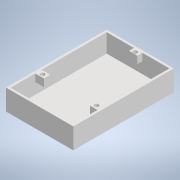
# Autodesk Inventor part: корпус
Saved by Autodesk Inventor 2022 (Build 260153000, 153)
## iProperties
Created: 2022-10-20
Part Number: корпус
Material: Типовые
Document SubType Name: Modeling
Designer: Robo0
Density: 1 g/cm^3
Appearance: По умолчанию
Author: Robo0
Autodesk Inventor part; units mm, degrees
ref_plane "YZ Plane" through (0, 0, 0) normal (1, 0, 0) x (0, 1, 0)
ref_plane "XZ Plane" through (0, 0, 0) normal (0, 1, 0) x (-1, 0, 0)
ref_plane "XY Plane" through (0, 0, 0) normal (0, 0, 1) x (1, 0, 0)
sketch "Эскиз1" plane through (0, 0, 0) normal (0, 1, 0) x (-1, 0, 0)
  line L0 (0, 0) -> (200, 0)
  line L1 (200, 0) -> (200, 200)
  line L2 (200, 200) -> (0, 200)
  line L3 (0, 200) -> (0, 0)
  dimension "d0" = 200
  dimension "d1" = 200
  constraints: 8 end point, 2 parallel, 1 horizontal, 1 perpendicular
  measures "d0" distance of L2.end L1.end
  measures "d1" distance of L1.end L0.end
extrude "Выдавливание1" add sketch "Эскиз1" along normal blind 3
sketch "Эскиз2" plane through (0, 3, 0) normal (0, 1, 0) x (1, 0, 0)
  line L0 (-200, 0) -> (-200, -200) projected
  line L1 (-200, -200) -> (0, -200) projected
  line L2 (0, -200) -> (0, 0) projected
  line L3 (0, 0) -> (-200, 0) projected
  line L4 (0, -200) -> (0, 0) projected
  line L5 (0, 0) -> (-90.778, 0)
  line L6 (-90.778, 0) -> (-90.778, -135.834)
  line L7 (-90.778, -135.834) -> (0, -135.834)
  line L8 (0, -135.834) -> (0, 0)
  constraints: 8 end point, 2 parallel, 1 horizontal, 1 perpendicular
extrude "Выдавливание2" cut sketch "Эскиз2" against normal blind 3 contours L3 L6 L7 L2 L1 L0
sketch "Эскиз3" plane through (0, 3, 0) normal (0, 1, 0) x (1, 0, 0)
  line L0 (-90.778, 0) -> (-90.778, -135.834) projected
  line L1 (-90.778, -135.834) -> (0, -135.834) projected
  line L2 (0, -135.834) -> (0, 0) projected
  line L3 (0, 0) -> (-90.778, 0) projected
  line L4 (-87.778, -132.834) -> (-3, -132.834)
  line L5 (-3, -132.834) -> (-3, -3)
  line L6 (-3, -3) -> (-87.778, -3)
  line L7 (-87.778, -3) -> (-87.778, -132.834)
  dimension "d6" = 3
  dimension "d7" = 3
  dimension "d8" = 3
  dimension "d9" = 3
  constraints: 8 end point, 2 parallel, 1 horizontal, 1 perpendicular
  measures "d6" distance between parallel lines of L0 L7
  measures "d7" distance between parallel lines of L6 L3
  measures "d8" distance between parallel lines of L2 L5
  measures "d9" distance between parallel lines of L1 L4
extrude "Выдавливание3" add sketch "Эскиз3" along normal blind 25
sketch "Эскиз4" plane through (0, 28, 0) normal (0, 1, 0) x (1, 0, 0)
  line L0 (-87.778, -3) -> (-3, -3) projected
  line L1 (-87.778, -132.834) -> (-87.778, -3) projected
  line L2 (-3, -3) -> (-3, -132.834) projected
  circle A0 centre (-81.778, -95.6228) radius 2.75
  circle A1 centre (-9, -95.6228) radius 2.75
  circle A2 centre (-45.389, -7) radius 2.75
  line L3 (-87.778, -99.5857) -> (-76.0264, -99.5857)
  line L4 (-76.0264, -99.5857) -> (-76.0264, -91)
  line L5 (-76.0264, -91) -> (-87.778, -91)
  line L6 (-87.778, -91) -> (-87.778, -99.5857)
  line L7 (-50.872, -3) -> (-39.6049, -3)
  line L8 (-39.6049, -3) -> (-39.6049, -9.75)
  line L9 (-39.6049, -9.75) -> (-50.872, -9.75)
  line L10 (-50.872, -9.75) -> (-50.872, -3)
  line L11 (-3, -91) -> (-13.2714, -91)
  line L12 (-13.2714, -91) -> (-13.2714, -100.2408)
  line L13 (-13.2714, -100.2408) -> (-3, -100.2408)
  line L14 (-3, -100.2408) -> (-3, -91)
  line L15 (-36, -90) -> (-62, -90) projected
  point P0 (0, 0)
  point P1 (-45.389, -9.75)
  point P2 (-3, -100.2408)
  dimension "d12" = 5.5
  dimension "d13" = 6
  dimension "d14" = 5.5
  dimension "d15" = 6
  dimension "d16" = 5.5
  dimension "d17" = 4
  dimension "d18" = 1
  dimension "d19" = 4.6227
  constraints: 24 end point, 6 parallel, 4 point on line, 3 centre point, 3 horizontal, 3 perpendicular
  measures "d12" diameter of A0
  measures "d13" distance from line of A0.centre L1
  measures "d14" diameter of A1
  measures "d15" distance from line of A1.centre L2
  measures "d16" diameter of A2
  measures "d17" distance from line of A2.centre L0
  measures "d18" distance between parallel lines of L5 L15
  measures "d19" distance from line of L5 A0.centre
extrude "Выдавливание4" add sketch "Эскиз4" against normal blind 10
sketch "Эскиз5" plane through (-90.778, 0, 0) normal (-1, 0, 0) x (0, 0, 1)
  point P0 (0, 0)
sketch "Эскиз6" plane through (-90.778, 0, 0) normal (-1, 0, 0) x (0, 0, 1)
  line L0 (123, 6.5) -> (123, 0.5) projected
  line L1 (129, 6.5) -> (123, 6.5) projected
  line L2 (129, 0.5) -> (129, 6.5) projected
  line L3 (129.6397, 6.975) -> (122.4748, 6.975)
  line L4 (122.4748, 6.975) -> (122.4748, 0.5)
  line L5 (122.4748, 0.5) -> (129.6397, 0.5)
  line L6 (129.6397, 0.5) -> (129.6397, 6.975)
  point P0 (0, 0)
  constraints: 8 end point, 2 parallel, 1 horizontal, 1 perpendicular
extrude "Выдавливание5" cut sketch "Эскиз6" against normal blind 10
